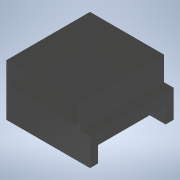
# Autodesk Inventor part: jetson_dummy
Saved by Autodesk Inventor 2021.3 (Build 253353010, 353A)
## iProperties
Created: 2021-07-26
Part Number: jetson_dummy
Material: Generisch
Document SubType Name: Modeling
Designer: Markus
Density: 1 g/cm^3
Appearance: Aluminium - poliert
Author: Markus
Autodesk Inventor part; units mm, degrees
ref_plane "YZ Plane" through (0, 0, 0) normal (1, 0, 0) x (0, 1, 0)
ref_plane "XZ Plane" through (0, 0, 0) normal (0, 1, 0) x (-1, 0, 0)
ref_plane "XY Plane" through (0, 0, 0) normal (0, 0, 1) x (1, 0, 0)
sketch "Skizze1" plane through (0, 0, 0) normal (0, 1, 0) x (-1, 0, 0)
  line L0 (0, 0) -> (105, 0)
  line L1 (105, 0) -> (105, -105)
  line L2 (105, -105) -> (0, -105)
  line L3 (0, -105) -> (0, 0)
  line L4 (0, -105) -> (93, -105)
  line L5 (93, -105) -> (93, 0)
  line L6 (93, 0) -> (0, 0)
  line L7 (0, 0) -> (0, -105)
  dimension "d0" = 105
  dimension "d1" = 105
  dimension "d2" = 93
  constraints: 16 end point, 4 parallel, 2 horizontal, 2 perpendicular, 1 point on line
  measures "d0" distance of L1.end L2.end
  measures "d1" distance of L0.end L1.end
  measures "d2" distance between parallel lines of L3 L5
extrude "Extrusion1" add sketch "Skizze1" along normal blind 45 contours L0 L5 L2 L3
sketch "Skizze2" plane through (0, 0, 0) normal (0, -1, 0) x (1, 0, 0)
  line L0 (0, -105) -> (-93, -105) projected
  line L1 (-93, -105) -> (12, -105)
  line L2 (12, -105) -> (12, 0)
  line L3 (12, 0) -> (-93, 0)
  line L4 (-93, 0) -> (-93, -105)
  line L5 (-93, -105) -> (-93, 0) projected
  line L6 (12, -105) -> (-93, -105)
  line L7 (-93, -105) -> (-93, -95)
  line L8 (-93, -95) -> (12, -95)
  line L9 (12, -95) -> (12, -105)
  line L10 (12, 0) -> (-93, 0)
  line L11 (-93, 0) -> (-93, -10)
  line L12 (-93, -10) -> (12, -10)
  line L13 (12, -10) -> (12, 0)
  point P0 (0, 0)
  point P1 (12, -10)
  point P2 (12, -95)
  dimension "d5" = 105
  dimension "d6" = 10
  dimension "d7" = 10
  constraints: 24 end point, 6 parallel, 3 horizontal, 3 perpendicular, 2 point on line, 1 horizontal alignment
  measures "d5" distance of L0.end L1.end
  measures "d6" distance between parallel lines of L1 L8
  measures "d7" distance between parallel lines of L3 L12
extrude "Extrusion2" add sketch "Skizze2" along normal blind 20 contours L0 L4 L8 L2 L1 | L4 L3 L2 L12
sketch "Skizze3" plane through (0, 0, 0) normal (0, 1, 0) x (1, 0, 0)
  line L0 (-93, 0) -> (0, 0) projected
  line L1 (0, 105) -> (12, 105) projected
  line L2 (0, 0) -> (12, 0)
  line L3 (12, 0) -> (12, 105)
  line L4 (12, 105) -> (0, 105)
  line L5 (0, 105) -> (0, 0)
  constraints: 8 end point, 2 parallel, 1 horizontal, 1 perpendicular
extrude "Extrusion3" add sketch "Skizze3" along normal blind 15
sketch "Skizze4" plane through (0, 45, -105) normal (0, 0, -1) x (-1, 0, 0)
  line L0 (93, -65) -> (93, 0) projected
  line L1 (0, 0) -> (93, 0) projected
  line L2 (0, -30) -> (0, 0) projected
  line L3 (-12, -30) -> (0, -30) projected
  line L4 (-12, -30) -> (-12, -65) projected
  line L5 (93, -65) -> (-12, -65) projected
  line L6 (3, -3) -> (90, -3)
  line L7 (90, -3) -> (90, -26)
  line L8 (90, -26) -> (3, -26)
  line L9 (3, -26) -> (3, -3)
  point P0 (0, -45)
  point P1 (46.5, -3)
  point P2 (46.5, 0)
  dimension "d12" = 3
  dimension "d13" = 3
  dimension "d14" = 23
  constraints: 8 end point, 2 midpoint, 2 parallel, 1 horizontal, 1 perpendicular, 1 vertical alignment
  measures "d12" distance between parallel lines of L2 L9
  measures "d13" distance between parallel lines of L1 L6
  measures "d14" distance between parallel lines of L6 L8
extrude "Extrusion4" cut sketch "Skizze4" against normal through all contours L6 L7 L8 L9
equation "\"d0\" = base_breite"
equation "\"d1\" = base_tiefe"
equation "\"d2\" = koerper_breite"
equation "\"d3\" = hoehe - fuss_höhe"
equation "\"d5\" = base_breite"
equation "\"d6\" = fuss_breite"
equation "\"d7\" = fuss_breite"
equation "\"d8\" = fuss_höhe"
equation "\"d10\" = PCI_hoehe"
equation "\"d12\" = koerper_wandstaerke"
equation "\"d13\" = koerper_wandstaerke"
equation "\"d14\" = kuehlöffnung"
equation "\"base_breite\" = 105"
equation "\"base_tiefe\" = 105"
equation "\"fuss_breite\" = 10"
equation "\"koerper_breite\" = 93"
equation "\"koerper_tiefe\" = 105"
equation "\"fuss_höhe\" = 20"
equation "\"hoehe\" = 65"
equation "\"PCI_hoehe\" = 15"
equation "\"koerper_wandstaerke\" = 3"
equation "\"kuehlöffnung\" = 23"
